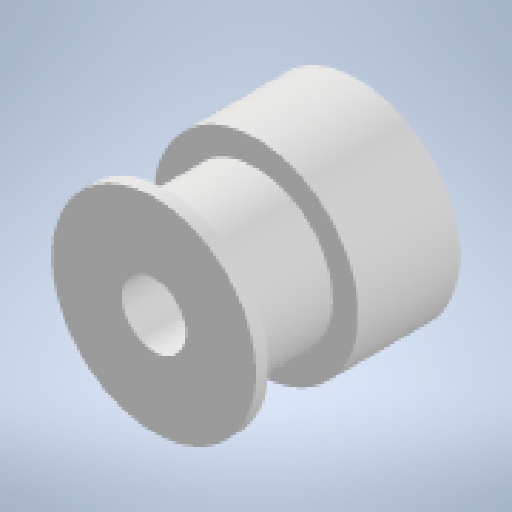
# Autodesk Inventor part: belt_gear_1
Saved by Autodesk Inventor 2024 (Build 280153000, 153)
## iProperties
Created: 2026-02-05
Part Number: belt_gear_1
Material: Generic
Document SubType Name: Modeling
Designer: SEMEN
Density: 1 g/cm^3
Appearance: Default
Author: SEMEN
Autodesk Inventor part; units mm, degrees
ref_plane "YZ Plane" through (0, 0, 0) normal (1, 0, 0) x (0, 1, 0)
ref_plane "XZ Plane" through (0, 0, 0) normal (0, 1, 0) x (-1, 0, 0)
ref_plane "XY Plane" through (0, 0, 0) normal (0, 0, 1) x (1, 0, 0)
sketch "Sketch1" plane through (0, 0, 0) normal (1, 0, 0) x (0, 1, 0)
  line L0 (0, 0) -> (8, 0)
  line L1 (8, 0) -> (8, 16)
  line L2 (8, 16) -> (0, 16)
  line L3 (0, 16) -> (0, 0)
  line L4 (8, 15) -> (2.5, 15)
  line L5 (8, 8) -> (2.5, 8)
  line L6 (6, 15) -> (6, 8)
  line L7 (2.5, 16) -> (2.5, 0)
  dimension "d7" = 8
  dimension "d8" = 16
  dimension "d9" = 1
  dimension "d10" = 7
  dimension "d11" = 6
  dimension "d12" = 2.5
  constraints: 16 end point, 6 point on line, 5 perpendicular, 2 midpoint, 2 parallel, 1 horizontal
  measures "d7" distance of L2.end L1.end
  measures "d8" distance of L1.end L0.end
  measures "d9" distance between parallel lines of L2 L4
  measures "d10" distance between parallel lines of L5 L4
  measures "d11" distance between parallel lines of L3 L6
  measures "d12" distance between parallel lines of L3 L7
revolve "Revolution1" add sketch "Sketch1" angle 360 about axis through (0, 0, 16) along (0, 0, 1) contours L7 L5 L1 L0 | L7 L4 L6 L5 | L2 L1 L4 L7
body "Solid1"
